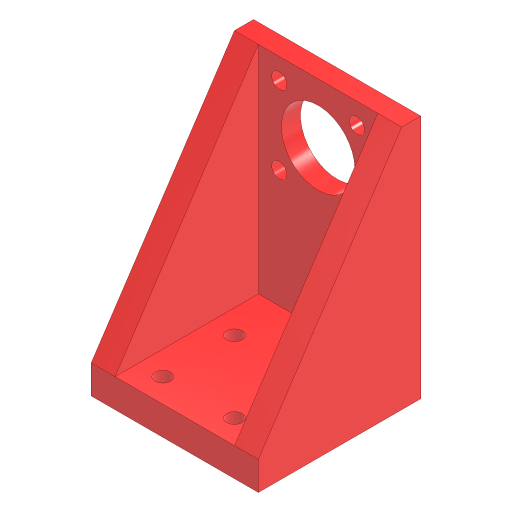
# Autodesk Inventor part: Part6
Saved by Autodesk Inventor 2024.3 (Build 283343000, 343)
## iProperties
Created: 2025-06-08
Part Number: Part6
Material: Generic
Document SubType Name: Modeling
Designer: MPA
Density: 1 g/cm^3
Appearance: Light Red
Author: MPA
## iProperties of the stored document Part6_3DPrint.ipt
Created: 2025-06-18
Part Number: Part6_3DPrint
Material: Generic
Document SubType Name: Modeling
Designer: MPA
Density: 1 g/cm^3
Appearance: Default
Author: MPA
Autodesk Inventor part; units mm, degrees
ref_plane "YZ Plane" through (0, 0, 0) normal (1, 0, 0) x (0, 1, 0)
ref_plane "XZ Plane" through (0, 0, 0) normal (0, 1, 0) x (-1, 0, 0)
ref_plane "XY Plane" through (0, 0, 0) normal (0, 0, 1) x (1, 0, 0)
sketch "Sketch1" plane through (0, 0, 0) normal (0, 0, 1) x (1, 0, 0)
  line L0 (-35, -25) -> (35, -25)
  line L1 (35, -25) -> (35, 25)
  line L2 (35, 25) -> (-35, 25)
  line L3 (-35, 25) -> (-35, -25)
  line L4 (-35, -25) -> (35, 25) construction
  line L5 (35, -25) -> (-35, 25) construction
  circle A0 centre (0, 0) radius 15.4
  dimension "d0" = 70
  dimension "d1" = 50
  dimension "d2" = 30.8
  constraints: 12 end point, 2 midpoint, 2 parallel, 1 centre point, 1 coincident, 1 horizontal, 1 perpendicular
  measures "d0" distance of L2.end L1.end
  measures "d1" distance of L1.end L0.end
  measures "d2" diameter of A0
extrude "Extrusion1" add sketch "Sketch1" along normal blind 8
sketch "Sketch2" plane through (0, 0, 8) normal (0, 0, 1) x (1, 0, 0)
  line L0 (35, -25) -> (35, 25) projected
  line L1 (35, 25) -> (-35, 25) projected
  line L2 (-35, 25) -> (-35, -25) projected
  line L3 (-35, -25) -> (35, -25) projected
  circle A0 centre (0, 0) radius 15.4 projected
  line L4 (16.25, -16.25) -> (-16.25, -16.25) construction
  line L5 (-16.25, -16.25) -> (-16.25, 16.25) construction
  line L6 (-16.25, 16.25) -> (16.25, 16.25) construction
  line L7 (16.25, 16.25) -> (16.25, -16.25) construction
  line L8 (16.25, -16.25) -> (-16.25, 16.25) construction
  line L9 (-16.25, -16.25) -> (16.25, 16.25) construction
  dimension "d5" = 32.5
  dimension "d6" = 32.5
  constraints: 12 end point, 4 coincident, 2 midpoint, 2 parallel, 1 horizontal, 1 perpendicular
  measures "d5" distance of L5.end L6.end
  measures "d6" distance of L4.end L5.end
hole "Hole1" at (-16.25, 16.25, 8) at (16.25, 16.25, 8) at (16.25, -16.25, 8) at (-16.25, -16.25, 8) direction (0, 0, -1) diameter 6.4 end through all clearance for "Hex Head Cap Screw ISO 24017" size "M6" standard "ISO"
sketch "Sketch3" plane through (0, 0, 8) normal (0, 0, 1) x (1, 0, 0)
  circle A0 centre (0, 0) radius 15.4 projected
  circle A1 centre (-16.25, -16.25) radius 3.2 projected
  circle A2 centre (16.25, -16.25) radius 3.2 projected
  circle A3 centre (16.25, 16.25) radius 3.2 projected
  circle A4 centre (-16.25, 16.25) radius 3.2 projected
  line L0 (35, -25) -> (35, 25) projected
  line L1 (35, 25) -> (-35, 25) projected
  line L2 (-35, 25) -> (-35, -25) projected
  line L3 (-35, -25) -> (35, -25) projected
  circle A5 centre (0, 0) radius 15.4 projected
  line L4 (-35, -25) -> (35, -25)
  line L5 (35, -25) -> (35, -77.5)
  line L6 (35, -77.5) -> (-35, -77.5)
  line L7 (-35, -77.5) -> (-35, -25)
  dimension "d14" = 77.5
  constraints: 8 end point, 2 parallel, 1 horizontal, 1 perpendicular, 1 vertical alignment
  measures "d14" distance from line of point (0, 0) L6
extrude "Extrusion2" add sketch "Sketch3" against normal up to surface (8 mm away) contours L5 L6 L7 L3
sketch "Sketch4" plane through (-35, 25, 0) normal (-1, 0, 0) x (0, 0, 1)
  line L0 (0, 0) -> (0, -102.5) projected
  line L1 (8, -102.5) -> (0, -102.5) projected
  line L2 (8, 0) -> (8, -102.5) projected
  line L3 (0, 0) -> (8, 0) projected
  line L4 (8, -102.5) -> (68, -102.5)
  line L5 (68, -102.5) -> (68, -90.5)
  line L6 (68, -90.5) -> (8, -90.5)
  line L7 (8, -90.5) -> (8, -102.5)
  line L8 (68, -90.5) -> (8, 0)
  point P0 (0, -25)
  dimension "d17" = 60
  dimension "d18" = 12
  constraints: 10 end point, 2 parallel, 1 horizontal, 1 perpendicular
  measures "d17" distance of L6.end L5.end
  measures "d18" distance of L5.end L4.end
extrude "Extrusion3" add sketch "Sketch4" against normal blind 10 contours L8 L6 L2 | L2 L6 L5 L4
mirror "Mirror1" about plane through (0, 0, 0) normal (1, 0, 0) of "Extrusion3"
sketch "Sketch5" plane through (-35, -77.5, 0) normal (0, -1, 0) x (1, 0, 0)
  line L0 (10, 68) -> (10, 8) projected
  line L1 (60, 68) -> (60, 8) projected
  line L2 (10, 8) -> (60, 8) projected
  line L3 (10, 68) -> (60, 68)
  point P0 (35, 0)
  constraints: 2 end point, 1 horizontal
extrude "Extrusion4" add sketch "Sketch5" against normal blind 12
sketch "Sketch6" plane through (-35, -65.5, 0) normal (0, 1, 0) x (1, 0, 0)
  line L0 (10, -68) -> (10, -8) projected
  line L1 (10, -68) -> (60, -68) projected
  line L2 (60, -8) -> (60, -68) projected
  line L3 (10, -8) -> (60, -8) projected
  line L4 (50, -18) -> (50, -58) construction
  line L5 (50, -58) -> (20, -58) construction
  line L6 (20, -58) -> (20, -18) construction
  line L7 (20, -18) -> (50, -18) construction
  point P0 (35, 0)
  dimension "d23" = 10
  constraints: 8 end point, 4 coincident, 3 other
  measures "d23" distance between parallel lines of L3 L7
hole "Hole2" at (-15, -65.5, 18) at (-15, -65.5, 58) at (15, -65.5, 18) at (15, -65.5, 58) direction (0, -1, 0) diameter 6.6 end through all clearance for "Hex Head Cap Screw ISO 24017" size "M6" standard "ISO"
move faces "Move1" translate (0, 0, 10) faces at (15.2655, -69.5, 21.2893) (-14.7345, -69.5, 21.2893)
body "Solid1"
